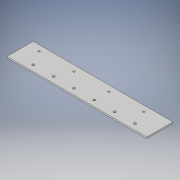
# Autodesk Inventor part: Rack-Elondo-Bracket
Saved by Autodesk Inventor 2019 (Build 230136000, 136)
## iProperties
Created: 2019-02-01
Part Number: Rack-Elondo-Bracket
Material: Generic
Document SubType Name: Modeling
Designer: bbramman
Density: 1 g/cm^3
Appearance: Default
Author: bbramman
Autodesk Inventor part; units mm, degrees
ref_plane "YZ Plane" through (0, 0, 0) normal (1, 0, 0) x (0, 1, 0)
ref_plane "XZ Plane" through (0, 0, 0) normal (0, 1, 0) x (-1, 0, 0)
ref_plane "XY Plane" through (0, 0, 0) normal (0, 0, 1) x (1, 0, 0)
sketch "Sketch1" plane through (0, 0, 0) normal (0, 1, 0) x (-1, 0, 0)
  line L0 (-152.4, 28.575) -> (152.4, 28.575)
  line L1 (152.4, 28.575) -> (152.4, -28.575)
  line L2 (152.4, -28.575) -> (-152.4, -28.575)
  line L3 (-152.4, -28.575) -> (-152.4, 28.575)
  line L4 (-152.4, 28.575) -> (152.4, -28.575) construction
  line L5 (152.4, 28.575) -> (-152.4, -28.575) construction
  point P0 (0, 0)
  dimension "d0" = 304.8
  dimension "d1" = 57.15
  constraints: 12 end point, 2 midpoint, 2 parallel, 1 horizontal, 1 perpendicular
  measures "d0" distance of L1.end L2.end
  measures "d1" distance of L0.end L1.end
extrude "Extrusion1" add sketch "Sketch1" along normal blind 3.175
sketch "Sketch2" plane through (0, 3.175, 0) normal (0, 1, 0) x (1, 0, 0)
  line L0 (152.4, 28.575) -> (-152.4, 28.575) projected
  line L1 (-152.4, -28.575) -> (152.4, -28.575) projected
  line L2 (0, -15.875) -> (-152.4, -15.875)
  line L3 (-152.4, 28.575) -> (-152.4, -28.575) projected
  line L4 (0, -15.875) -> (152.4, -15.875)
  line L5 (0, 15.875) -> (-152.4, 15.875)
  line L6 (0, 15.875) -> (152.4, 15.875)
  line L7 (152.4, -28.575) -> (152.4, 28.575) projected
  line L8 (-152.4, -15.875) -> (-107.95, -15.875)
  line L9 (-107.95, -15.875) -> (-63.5, -15.875)
  line L10 (-63.5, -15.875) -> (-19.05, -15.875)
  line L11 (-19.05, -15.875) -> (25.4, -15.875)
  line L12 (25.4, -15.875) -> (69.85, -15.875)
  line L13 (69.85, -15.875) -> (114.3, -15.875)
  line L14 (-152.4, 15.875) -> (-127, 15.875)
  line L15 (-127, 15.875) -> (-50.8, 15.875)
  line L16 (-50.8, 15.875) -> (25.4, 15.875)
  line L17 (25.4, 15.875) -> (101.6, 15.875)
  point P0 (0, 0)
  dimension "d8" = 44.45
  dimension "d9" = 44.45
  dimension "d10" = 44.45
  dimension "d11" = 44.45
  dimension "d12" = 44.45
  dimension "d13" = 44.45
  dimension "d14" = 25.4
  dimension "d15" = 76.2
  dimension "d16" = 76.2
  dimension "d17" = 76.2
  constraints: 28 end point, 15 point on line, 10 coincident, 2 horizontal
  measures "d8" distance of L2.end L8.end
  measures "d9" distance of L8.end L9.end
  measures "d10" distance of L9.end L10.end
  measures "d11" distance of L10.end L11.end
  measures "d12" distance of L11.end L12.end
  measures "d13" distance of L12.end L13.end
  measures "d14" distance of L5.end L14.end
  measures "d15" distance of L14.end L15.end
  measures "d16" distance of L15.end L16.end
  measures "d17" distance of L16.end L17.end
hole "Hole1" at (-107.95, 3.175, 15.875) at (-63.5, 3.175, 15.875) at (-19.05, 3.175, 15.875) at (25.4, 3.175, 15.875) at (69.85, 3.175, 15.875) at (114.3, 3.175, 15.875) direction (0, -1, 0) diameter 5.1054 end through all clearance for "Flat Head Machine Screw (82)" size "#10" standard "Ansi Unified Screw Threads"
sketch "Sketch3" plane through (0, 3.175, 0) normal (0, 1, 0) x (1, 0, 0)
  line L0 (152.4, 28.575) -> (-152.4, 28.575)
  line L1 (-152.4, -28.575) -> (152.4, -28.575)
  line L2 (0, -15.875) -> (-152.4, -15.875)
  line L3 (-152.4, 28.575) -> (-152.4, -28.575)
  line L4 (0, -15.875) -> (152.4, -15.875)
  line L5 (0, 15.875) -> (-152.4, 15.875)
  line L6 (0, 15.875) -> (152.4, 15.875)
  line L7 (152.4, -28.575) -> (152.4, 28.575)
  line L8 (-152.4, -15.875) -> (-107.95, -15.875)
  line L9 (-107.95, -15.875) -> (-63.5, -15.875)
  line L10 (-63.5, -15.875) -> (-19.05, -15.875)
  line L11 (-19.05, -15.875) -> (25.4, -15.875)
  line L12 (25.4, -15.875) -> (69.85, -15.875)
  line L13 (69.85, -15.875) -> (114.3, -15.875)
  line L14 (-152.4, 15.875) -> (-127, 15.875)
  line L15 (-127, 15.875) -> (-50.8, 15.875)
  line L16 (-50.8, 15.875) -> (25.4, 15.875)
  line L17 (25.4, 15.875) -> (101.6, 15.875)
  point P0 (0, 0)
  point P1 (0, 0)
  dimension "d25" = 44.45
  dimension "d26" = 44.45
  dimension "d27" = 44.45
  dimension "d28" = 44.45
  dimension "d29" = 44.45
  dimension "d30" = 44.45
  dimension "d31" = 25.4
  dimension "d32" = 76.2
  dimension "d33" = 76.2
  dimension "d34" = 76.2
  constraints: 36 end point, 15 point on line, 10 coincident, 2 horizontal
  measures "d25" distance of L2.end L8.end
  measures "d26" distance of L8.end L9.end
  measures "d27" distance of L9.end L10.end
  measures "d28" distance of L10.end L11.end
  measures "d29" distance of L11.end L12.end
  measures "d30" distance of L12.end L13.end
  measures "d31" distance of L5.end L14.end
  measures "d32" distance of L14.end L15.end
  measures "d33" distance of L15.end L16.end
  measures "d34" distance of L16.end L17.end
hole "Hole2" at (-127, 3.175, -15.875) at (-50.8, 3.175, -15.875) at (25.4, 3.175, -15.875) at (101.6, 3.175, -15.875) direction (0, -1, 0) diameter 3.81 end through all clearance for "Flat Head Machine Screw (82)" size "#6" standard "Ansi Unified Screw Threads"
body "Solid1"
